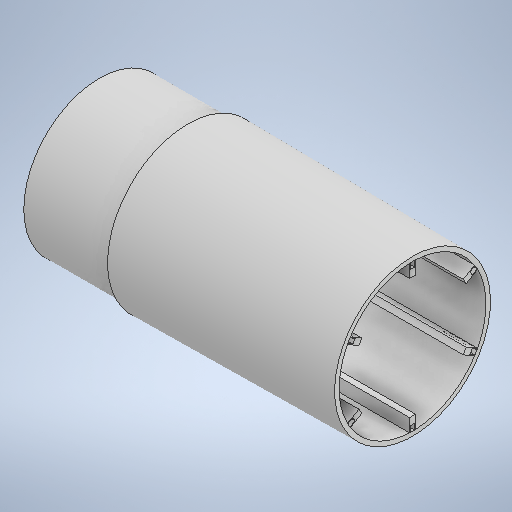
# Autodesk Inventor part: Nosecone(finale)
Saved by Autodesk Inventor 2025 (Build 290162000, 162)
## iProperties
Created: 2024-06-04
Part Number: Nosecone(finale)
Material: Generic
Document SubType Name: Sheet Metal
Designer: agnes
Density: 1 g/cm^3
Sheet Metal Rule: Default_mm
Appearance: Default
Author: agnes
Autodesk Inventor part; units mm, degrees
ref_plane "XZ Plane" through (0, 0, 0) normal (0, 1, 0) x (-1, 0, 0)
ref_plane "XY Plane" through (0, 0, 0) normal (0, 0, 1) x (1, 0, 0)
sketch "Reinforcment" plane through (0, 0, 0) normal (0, 0, 1) x (1, 0, 0)
  line L0 (0, 0) -> (-150, 0)
  line L1 (-150, 0) -> (-150, 51.5)
  line L2 (-150, 51.5) -> (0, 50)
  line L3 (-154.0291, 0.0806) -> (-152.94, 54.5296)
  line L4 (-152.94, 54.5296) -> (0, 53.0001)
  line L5 (-150, 0) -> (-154.0291, 0.0806)
  line L6 (0, 50) -> (0, 53.0001)
  dimension "d1" = 50
  dimension "d2" = 51.5
  dimension "d3" = 3
  constraints: 14 end point, 2 vertical, 1 horizontal, 1 perpendicular
  measures "d1" distance of L0.start L2.end
  measures "d2" distance of L0.end L1.end
  measures "d3" distance between parallel lines of L2 L4
revolve "Revolution1" add sketch "Reinforcment" angle 360 about axis through (0, 0, 0) along (-1, 0, 0)
sketch "Sketch2" plane through (0, 0, 0) normal (1, 0, 0) x (0, 0, -1)
  circle A0 centre (0, 0) radius 50 projected
  line L0 (0, 50) -> (2, 50)
  line L1 (2, 50) -> (2, 41)
  line L2 (2, 41) -> (0, 41)
  line L3 (0, 50) -> (-2, 50)
  line L4 (-2, 50) -> (-2, 41)
  line L5 (-2, 41) -> (0, 41)
  line L6 (-43.3013, 25) -> (-42.3013, 26.7321)
  line L7 (-42.3013, 26.7321) -> (-34.507, 22.2321)
  line L8 (-34.507, 22.2321) -> (-35.507, 20.5)
  line L9 (-43.3013, 25) -> (-44.3013, 23.2679)
  line L10 (-44.3013, 23.2679) -> (-36.507, 18.7679)
  line L11 (-36.507, 18.7679) -> (-35.507, 20.5)
  line L12 (-43.3013, -25) -> (-44.3013, -23.2679)
  line L13 (-44.3013, -23.2679) -> (-36.507, -18.7679)
  line L14 (-36.507, -18.7679) -> (-35.507, -20.5)
  line L15 (-43.3013, -25) -> (-42.3013, -26.7321)
  line L16 (-42.3013, -26.7321) -> (-34.507, -22.2321)
  line L17 (-34.507, -22.2321) -> (-35.507, -20.5)
  line L18 (0, -50) -> (-2, -50)
  line L19 (-2, -50) -> (-2, -41)
  line L20 (-2, -41) -> (0, -41)
  line L21 (0, -50) -> (2, -50)
  line L22 (2, -50) -> (2, -41)
  line L23 (2, -41) -> (0, -41)
  line L24 (43.3013, -25) -> (42.3013, -26.7321)
  line L25 (42.3013, -26.7321) -> (34.507, -22.2321)
  line L26 (34.507, -22.2321) -> (35.507, -20.5)
  line L27 (43.3013, -25) -> (44.3013, -23.2679)
  line L28 (44.3013, -23.2679) -> (36.507, -18.7679)
  line L29 (36.507, -18.7679) -> (35.507, -20.5)
  line L30 (43.3013, 25) -> (44.3013, 23.2679)
  line L31 (44.3013, 23.2679) -> (36.507, 18.7679)
  line L32 (36.507, 18.7679) -> (35.507, 20.5)
  line L33 (43.3013, 25) -> (42.3013, 26.7321)
  line L34 (42.3013, 26.7321) -> (34.507, 22.2321)
  line L35 (34.507, 22.2321) -> (35.507, 20.5)
  point P0 (44.2666, 23.2479)
  point P1 (42.2666, 26.712)
  point P2 (42.2666, -26.712)
  point P3 (44.2666, -23.2479)
  point P4 (0, -41)
  point P5 (-2, -49.96)
  point P6 (2, -49.96)
  point P7 (-44.2666, -23.2479)
  point P8 (-42.2666, -26.712)
  point P9 (-42.2666, 26.712)
  point P10 (-44.2666, 23.2479)
  point P11 (2, 49.96)
  point P12 (-2, 49.96)
  dimension "d5" = 2
  dimension "d6" = 9
  dimension "d7" = 2
  dimension "d10" = 360
  constraints: 72 end point, 6 point on line, 2 horizontal, 2 parallel, 2 perpendicular, 81 other
  measures "d5" distance of L1.end L2.end
  measures "d6" distance of L0.end L1.end
  measures "d7" distance of L5.end L4.end
extrude "Extrusion1" add sketch "Sketch2" against normal up to next contours L31 L32 L35 L34 A0 | A0 L25 L26 L29 L28 | L1 L2 L5 L4 A0 | A0 L19 L20 L23 L22 | L7 L8 L11 L10 A0 | A0 L13 L14 L17 L16
sketch "Sketch3" plane through (0, 0, 0) normal (1, 0, 0) x (0, 0, -1)
  circle A0 centre (0, 0) radius 53.8081
  circle A1 centre (0, 0) radius 50
  line L0 (0, 50) -> (1.5, 50)
  line L1 (1.5, 50) -> (1.5, 46)
  line L2 (1.5, 46) -> (0, 46)
  line L3 (0, 50) -> (-1.5, 50)
  line L4 (-1.5, 50) -> (-1.5, 46)
  line L5 (-1.5, 46) -> (0, 46)
  line L6 (-43.3013, 25) -> (-42.5513, 26.299)
  line L7 (-42.5513, 26.299) -> (-39.0872, 24.299)
  line L8 (-39.0872, 24.299) -> (-39.8372, 23)
  line L9 (-43.3013, 25) -> (-44.0513, 23.701)
  line L10 (-44.0513, 23.701) -> (-40.5872, 21.701)
  line L11 (-40.5872, 21.701) -> (-39.8372, 23)
  line L12 (-43.3013, -25) -> (-44.0513, -23.701)
  line L13 (-44.0513, -23.701) -> (-40.5872, -21.701)
  line L14 (-40.5872, -21.701) -> (-39.8372, -23)
  line L15 (-43.3013, -25) -> (-42.5513, -26.299)
  line L16 (-42.5513, -26.299) -> (-39.0872, -24.299)
  line L17 (-39.0872, -24.299) -> (-39.8372, -23)
  line L18 (0, -50) -> (-1.5, -50)
  line L19 (-1.5, -50) -> (-1.5, -46)
  line L20 (-1.5, -46) -> (0, -46)
  line L21 (0, -50) -> (1.5, -50)
  line L22 (1.5, -50) -> (1.5, -46)
  line L23 (1.5, -46) -> (0, -46)
  line L24 (43.3013, -25) -> (42.5513, -26.299)
  line L25 (42.5513, -26.299) -> (39.0872, -24.299)
  line L26 (39.0872, -24.299) -> (39.8372, -23)
  line L27 (43.3013, -25) -> (44.0513, -23.701)
  line L28 (44.0513, -23.701) -> (40.5872, -21.701)
  line L29 (40.5872, -21.701) -> (39.8372, -23)
  line L30 (43.3013, 25) -> (44.0513, 23.701)
  line L31 (44.0513, 23.701) -> (40.5872, 21.701)
  line L32 (40.5872, 21.701) -> (39.8372, 23)
  line L33 (43.3013, 25) -> (42.5513, 26.299)
  line L34 (42.5513, 26.299) -> (39.0872, 24.299)
  line L35 (39.0872, 24.299) -> (39.8372, 23)
  point P0 (-42.5318, 26.2878)
  point P1 (-44.0318, 23.6897)
  point P2 (-44.0318, -23.6897)
  point P3 (-42.5318, -26.2878)
  point P4 (0, -46)
  point P5 (-1.5, -49.9775)
  point P6 (1.5, -49.9775)
  point P7 (42.5318, -26.2878)
  point P8 (44.0318, -23.6897)
  point P9 (44.0318, 23.6897)
  point P10 (42.5318, 26.2878)
  point P11 (1.5, 49.9775)
  point P12 (-1.5, 49.9775)
  dimension "d32" = 1.5
  dimension "d33" = 4
  dimension "d34" = 1.5
  dimension "d37" = 360
  constraints: 72 end point, 6 point on line, 2 coincident, 2 horizontal, 2 parallel, 2 perpendicular, 1 centre point, 82 other
  measures "d32" distance of L1.end L2.end
  measures "d33" distance of L0.end L1.end
  measures "d34" distance of L5.end L4.end
extrude "Extrusion2" cut sketch "Sketch3" against normal blind 20 contours L31 L32 L35 L34 A1 | A1 L25 L26 L29 L28 | L1 L2 L5 L4 A1 | A1 L19 L20 L23 L22 | L7 L8 L11 L10 A1 | A1 L13 L14 L17 L16
ref_plane "Work Plane1" through (-153, 0, 0) normal (1, 0, 0) x (0, 1, 0)
sketch "Sketch5" plane through (-153, 0, 0) normal (1, 0, 0) x (0, 1, 0)
  circle A0 centre (0, 0) radius 51.5
  circle A1 centre (0, 0) radius 49.875
  dimension "d28" = 103
  dimension "d29" = 99.75
  constraints: 2 centre point, 2 coincident
  measures "d28" diameter of A0
  measures "d29" diameter of A1
extrude "Extrusion4" add sketch "Sketch5" against normal blind 60
equation "\"BendRadius\" = Thickness"
equation "\"BendReliefWidth\" = Thickness"
equation "\"BendReliefDepth\" = 0.5 * Thickness"
equation "\"CornerReliefSize\" = 4 * Thickness"
equation "\"MinimumRemnant\" = 2 * Thickness"
equation "\"TransitionRadius\" = BendRadius"
equation "\"JacobiRadiusSize\" = BendRadius"
equation "\"GapSize\" = Thickness"
equation "\"Thickness\" = 0.5"
body "Solid1"
